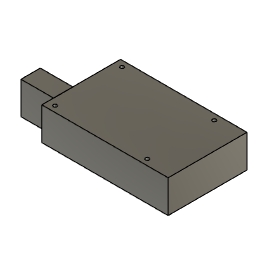
Amplifier (Autodesk Fusion 360 design; units mm, degrees)
Autodesk Fusion 360 part; units mm, degrees
sketch "Esquisse5" plane through (0, 0, 0) normal (0, 0, 1) x (1, 0, 0)
  line L0 (42.5, 26.5) -> (-42.5, 26.5)
  line L1 (-42.5, 26.5) -> (-42.5, -26.5)
  line L2 (-42.5, -26.5) -> (42.5, -26.5)
  line L3 (42.5, -26.5) -> (42.5, 26.5)
  circle A0 centre (-37.5, 22.5) radius 1.25
  circle A1 centre (24.5, 22.5) radius 1.25
  circle A2 centre (-37.5, -22.5) radius 1.25
  circle A3 centre (24.5, -22.5) radius 1.25
  dimension "d39" = 85
  dimension "d40" = 53
  dimension "d41" = 2.5
  dimension "d42" = 2.5
  dimension "d43" = 2.5
  dimension "d44" = 2.5
  dimension "d45" = 5
  dimension "d46" = 62
  dimension "d47" = 4
  dimension "d48" = 4
  dimension "d49" = 4
  dimension "d50" = 4
  dimension "d51" = 62
  dimension "d52" = 5
  constraint horizontal L0
  constraint perpendicular L0 L1
  constraint parallel L0 L2
  constraint parallel L1 L3
  measures "d39" distance of L1.end L2.end
  measures "d40" distance of L0.end L1.end
  measures "d41" diameter of A0
  measures "d42" diameter of A1
  measures "d43" diameter of A2
  measures "d44" diameter of A3
  measures "d45" distance of L1 A0.centre
  measures "d46" horizontal distance of A0.centre A1.centre
  measures "d47" distance of L0 A0.centre
  measures "d48" distance of L0 A1.centre
  measures "d49" distance of L2 A2.centre
  measures "d50" distance of L2 A3.centre
  measures "d51" distance of A2.centre A3.centre
  measures "d52" distance of L1 A2.centre
extrude "Extrusion10" add sketch "Esquisse5" along normal blind 22
sketch "Esquisse6" plane through (-42.5, 0, 0) normal (-1, 0, 0) x (0, -1, 0)
  line L0 (-26.5, 0) -> (26.5, 0)
  line L1 (26.5, 0) -> (26.5, 22)
  line L2 (26.5, 22) -> (-26.5, 22)
  line L3 (-26.5, 22) -> (-26.5, 0)
  line L4 (5.5, 21.893) -> (18.5, 21.893)
  line L5 (18.5, 21.893) -> (18.5, 0.0802)
  line L6 (18.5, 0.0802) -> (5.5, 0.0802)
  line L7 (5.5, 0.0802) -> (5.5, 21.893)
  dimension "d55" = 32
  dimension "d56" = 45
  constraint horizontal L4
  constraint vertical L5
  constraint horizontal L6
  constraint vertical L7
  measures "d55" distance of L3 L7
  measures "d56" distance of L3 L5
extrude "Extrusion11" add sketch "Esquisse6" along normal blind 22 contours L4 L5 L6 L7
